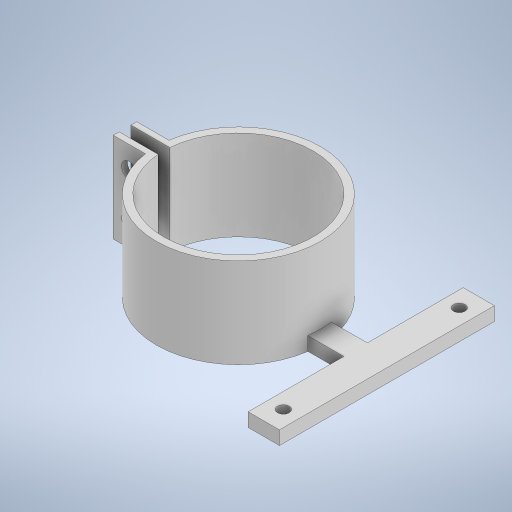
# Autodesk Inventor part: Bracket kamera
Saved by Autodesk Inventor 2024 (Build 280153000, 153)
## iProperties
Created: 2023-11-02
Part Number: Bracket kamera
Material: Generic
Document SubType Name: Modeling
Designer: lazy1
Density: 1 g/cm^3
Appearance: Default
Author: lazy1
Autodesk Inventor part; units mm, degrees
ref_plane "YZ Plane" through (0, 0, 0) normal (1, 0, 0) x (0, 1, 0)
ref_plane "XZ Plane" through (0, 0, 0) normal (0, 1, 0) x (-1, 0, 0)
ref_plane "XY Plane" through (0, 0, 0) normal (0, 0, 1) x (1, 0, 0)
sketch "Sketch1" plane through (0, 0, 0) normal (0, 1, 0) x (-1, 0, 0)
  arc A0 (16.9801, 0.913) -> (16.9801, -0.913) centre (-4, 0) ccw
  circle A1 centre (-4, 0) radius 21
  circle A2 centre (-4, 0) radius 19.1
  line L0 (17, 0) -> (25, 0)
  line L1 (25, 0) -> (25, -1.5)
  line L2 (25, -1.5) -> (15.041, -1.5)
  line L3 (25, 0) -> (25, 1.5)
  line L4 (25, 1.5) -> (15.041, 1.5)
  line L5 (25, -1.5) -> (25, -3)
  line L6 (25, -3) -> (14.8629, -3)
  line L7 (25, 1.5) -> (25, 3)
  line L8 (25, 3) -> (14.8629, 3)
  line L9 (-25, 0) -> (-34, 0)
  line L10 (-34, 0) -> (-42, 0)
  line L11 (-42, 0) -> (-42, 27.5)
  line L12 (-42, 27.5) -> (-34, 27.5)
  line L13 (-34, 27.5) -> (-34, 0)
  line L14 (-42, 0) -> (-42, -27.5)
  line L15 (-42, -27.5) -> (-34, -27.5)
  line L16 (-34, -27.5) -> (-34, 0)
  line L17 (-29.5, 0) -> (-29.5, 3)
  line L18 (-29.5, 3) -> (-24.7846, 3)
  line L19 (-29.5, 3) -> (-34, 3)
  line L20 (-29.5, 0) -> (-29.5, -3)
  line L21 (-29.5, -3) -> (-24.7846, -3)
  line L22 (-29.5, -3) -> (-34, -3)
  point P0 (-22.9783, -26)
  point P1 (16.7846, 3)
  point P2 (16.7846, -3)
  point P3 (-24.7846, 3)
  dimension "d8" = 38.2
  dimension "d9" = 8
  dimension "d10" = 1.5
  dimension "d11" = 1.5
  dimension "d12" = 1.5
  dimension "d13" = 1.5
  dimension "d31" = 21
  dimension "d60" = 9
  dimension "d61" = 8
  dimension "d62" = 27.5
  dimension "d63" = 27.5
  dimension "d64" = 3
  dimension "d65" = 3
  constraints: 46 end point, 12 perpendicular, 11 point on circle, 11 point on line, 3 centre point, 2 coincident, 2 horizontal, 1 midpoint, 1 vertical
  measures "d8" diameter of A2
  measures "d9" distance of L0.start L0.end
  measures "d10" distance of L0.end L1.end
  measures "d11" distance of L0.end L3.end
  measures "d12" distance of L1.end L5.end
  measures "d13" distance of L3.end L7.end
  measures "d31" radius of A0
  measures "d60" distance of L9.start L9.end
  measures "d61" distance of L9.end L10.end
  measures "d62" distance of L10.end L11.end
  measures "d63" distance of L10.end L14.end
  measures "d64" distance of L17.start L17.end
  measures "d65" distance of L17.start L20.end
extrude "Extrusion1" add sketch "Sketch1" along normal blind 23 contours A0 L8 A2 L6 | A0 L9 L17 L18 | A0 L21 L20 L9 | L8 L7 L4 A0 | A0 L4 A2 L8 | L17 L9 L13 L19 | L20 L22 L16 L9 | L13 L10 L11 L12 | L6 A2 L2 A0 | A0 L2 L5 L6 | L16 L15 L14 L10
sketch "Sketch4" plane through (-16.7846, 0, -3) normal (0, 0, -1) x (-1, 0, 0)
  line L0 (0, 0) -> (-41.5692, 0) projected
  line L1 (8.2154, 0) -> (8.2154, 23) projected
  line L2 (0, 0) -> (8.2154, 0)
  line L3 (8.2154, 0) -> (8.2154, 23)
  line L4 (8.2154, 23) -> (0, 23)
  line L5 (0, 23) -> (0, 0)
  line L6 (0, 11.5) -> (8.2154, 11.5)
  line L7 (4.1077, 11.5) -> (4.1077, 23)
  line L8 (4.1077, 11.5) -> (4.1077, 0)
  point P0 (-16.7846, 0)
  point P1 (4.1077, 5.75)
  point P2 (4.1077, 17.25)
  constraints: 14 end point, 7 midpoint, 2 parallel, 1 horizontal, 1 perpendicular
hole "Hole2" at (-20.8923, 5.75, -3) at (-20.8923, 17.25, -3) direction (0, 0, 1) diameter 4 depth 8 tip angle 118
sketch "Sketch8" plane through (0, 23, 0) normal (0, 1, 0) x (1, 0, 0)
  line L0 (34, 3) -> (24.7846, 3) projected
  line L1 (34, 3) -> (24.7846, 3)
  line L2 (34, 27.5) -> (34, 3) projected
  line L3 (34, 3) -> (34, 27.5)
  line L4 (42, -27.5) -> (42, 27.5) projected
  line L5 (34, 27.5) -> (42, 27.5)
  line L6 (42, 27.5) -> (42, -27.5)
  line L7 (42, -27.5) -> (34, -27.5)
  line L8 (24.7846, -3) -> (34, -3) projected
  line L9 (34, -27.5) -> (34, -3)
  line L10 (34, -3) -> (24.7846, -3)
  arc A0 (24.7846, 3) -> (-16.7846, 3) centre (4, 0) ccw projected
  line L11 (4, 21) -> (4, 0)
  circle A1 centre (4, 0) radius 21
  point P0 (0, 0)
  point P1 (24.7846, 3)
  point P2 (24.7846, -3)
  dimension "d78" = 42
  constraints: 16 end point, 3 collinear, 3 perpendicular, 2 vertical, 1 centre point, 1 coincident, 1 point on circle, 1 point on line
  measures "d78" diameter of A1
extrude "Extrusion5" cut sketch "Sketch8" against normal blind 19.5 contours L2 L5 L4 L7 L9 L8 A1 L0
sketch "Sketch9" plane through (0, 3.5, 0) normal (0, 1, 0) x (1, 0, 0)
  line L0 (34, 3) -> (34, 27.5) projected
  line L1 (34, -3) -> (34, 3)
  line L2 (34, 3) -> (34, 0)
  line L3 (42, 27.5) -> (42, -27.5) projected
  line L4 (42, 0) -> (34, 0)
  line L5 (38, 0) -> (38, -22.5)
  line L6 (38, 0) -> (38, 22.5)
  point P0 (0, 0)
  dimension "d69" = 22.5
  dimension "d70" = 22.5
  constraints: 10 end point, 3 midpoint, 2 coincident, 2 vertical, 1 parallel, 1 perpendicular
  measures "d69" distance of L5.start L5.end
  measures "d70" distance of L5.start L6.end
hole "Hole4" at (38, 3.5, -22.5) at (38, 3.5, 22.5) direction (0, -1, 0) diameter 3 depth 8 tip angle 118
body "Solid1"
